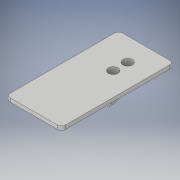
# Autodesk Inventor part: top
Saved by Autodesk Inventor 2017.3 (Build 213257000, 257)
## iProperties
Part Number: top
Material: Generisch
Document SubType Name: Modeling
Designer: Enno
Density: 1 g/cm^3
Appearance: Vorgabe
Author: Enno
Autodesk Inventor part; units mm, degrees
ref_plane "YZ Plane" through (0, 0, 0) normal (1, 0, 0) x (0, 1, 0)
ref_plane "XZ Plane" through (0, 0, 0) normal (0, 1, 0) x (-1, 0, 0)
ref_plane "XY Plane" through (0, 0, 0) normal (0, 0, 1) x (1, 0, 0)
sketch "Skizze1" plane through (0, 0, 0) normal (0, 0, 1) x (1, 0, 0)
  line L0 (0, 0) -> (29, 0)
  line L1 (29, 0) -> (29, 59)
  line L2 (29, 59) -> (0, 59)
  line L3 (0, 59) -> (0, 0)
  dimension "d0" = 29
  dimension "d1" = 59
  constraints: 8 end point, 2 parallel, 1 horizontal, 1 perpendicular
  measures "d0" distance of L1.end L2.end
  measures "d1" distance of L0.end L1.end
extrude "Extrusion1" add sketch "Skizze1" against normal blind 2
sketch "Skizze2" plane through (0, 0, -2) normal (0, 0, -1) x (-1, 0, 0)
  line L0 (-2, 2) -> (-27, 2)
  line L1 (-27, 2) -> (-27, 57)
  line L2 (-27, 57) -> (-2, 57)
  line L3 (-2, 57) -> (-2, 2)
  line L4 (0, 0) -> (0, 59) construction
  line L5 (-29, 0) -> (0, 0) construction
  point P0 (-2, 29.5)
  point P1 (0, 29.5)
  point P2 (-14.5, 2)
  point P3 (-14.5, 0)
  dimension "d4" = 2
  dimension "d5" = 2
  constraints: 8 end point, 4 midpoint, 2 parallel, 1 horizontal, 1 horizontal alignment, 1 perpendicular, 1 vertical alignment
  measures "d4" distance between parallel lines of L5 L0
  measures "d5" distance between parallel lines of L4 L3
extrude "Extrusion2" add sketch "Skizze2" along normal blind 2
sketch "Skizze3" plane through (0, 0, -4) normal (0, 0, -1) x (-1, 0, 0)
  circle A0 centre (-16.8, 39.4) radius 2.5
  line L0 (-29, 0) -> (0, 0) projected
  line L1 (-2, 2) -> (-2, 57) projected
  line L2 (-27, 57) -> (-27, 2) projected
  circle A1 centre (-16.8, 47.02) radius 2.5
  dimension "d8" = 5
  dimension "d9" = 39.4
  dimension "d11" = 10.2
  dimension "d12" = 5
  dimension "d13" = 7.62
  constraints: 2 centre point, 1 vertical alignment
  measures "d8" diameter of A0
  measures "d9" distance from line of L0 A0.centre
  measures "d11" distance from line of L2 A0.centre
  measures "d12" diameter of A1
  measures "d13" distance of A0.centre A1.centre
extrude "Extrusion3" cut sketch "Skizze3" against normal through all
fillet "Rundung1" radius 1 4 edges at (14.5, 57, -4) (27, 29.5, -4) (2, 29.5, -4) (14.5, 2, -4)
fillet "Rundung2" radius 2 4 edges at (0, 59, -1) (0, 0, -1) (29, 59, -1) (29, 0, -1)
sketch "Skizze4" plane through (0, 0, -4) normal (0, 0, -1) x (-1, 0, 0)
  line L0 (-24.5, 31.8) -> (-4.5, 31.8)
  line L1 (-4.5, 31.8) -> (-4.5, 35.3)
  line L2 (-4.5, 35.3) -> (-24.5, 35.3)
  line L3 (-24.5, 35.3) -> (-24.5, 31.8)
  line L4 (-27, 2) -> (-2, 2) projected
  point P0 (0, 0)
  point P1 (-14.5, 31.8)
  point P2 (-14.5, 2)
  dimension "d18" = 20
  dimension "d19" = 3.5
  dimension "d20" = 29.8
  constraints: 8 end point, 2 midpoint, 2 parallel, 1 horizontal, 1 perpendicular, 1 vertical alignment
  measures "d18" distance between parallel lines of L1 L3
  measures "d19" distance between parallel lines of L2 L0
  measures "d20" distance between parallel lines of L4 L0
extrude "Extrusion4" add sketch "Skizze4" along normal blind 6.01
sketch "Skizze6" plane through (4.5, 31.8, -4) normal (0, -1, 0) x (1, 0, 0)
  line L0 (0, -6.01) -> (2.5, -6.01)
  line L1 (2.5, -6.01) -> (0, -2)
  line L2 (0, -2) -> (0, -6.01)
  line L3 (20, 0) -> (0, 0) construction
  line L4 (10, 0) -> (10, 6.9424) construction
  line L5 (20, -6.01) -> (17.5, -6.01)
  line L6 (17.5, -6.01) -> (20, -2)
  line L7 (20, -2) -> (20, -6.01)
  point P0 (-4.5, 4)
  dimension "d29" = 2
  dimension "d30" = 2.5
  dimension "d31" = 4.01
  constraints: 14 end point, 3 symmetric about line, 1 midpoint, 1 perpendicular, 1 vertical
  measures "d29" distance from line of L3 L1.end
  measures "d30" distance of L0.start L0.end
  measures "d31" distance of L1.end L0.start
extrude "Extrusion5" cut sketch "Skizze6" against normal up to surface (3.5 mm away)
